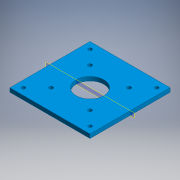
# Autodesk Inventor part: Part3
Saved by Autodesk Inventor 2016 (Build 200138000, 138)
## iProperties
Created: 2018-01-17
Part Number: Part3
Material: Generic
Document SubType Name: Modeling
Designer: student
Density: 1 g/cm^3
Appearance: Default
Author: student
Autodesk Inventor part; units mm, degrees
ref_plane "YZ Plane" through (0, 0, 0) normal (1, 0, 0) x (0, 1, 0)
ref_plane "XZ Plane" through (0, 0, 0) normal (0, 1, 0) x (-1, 0, 0)
ref_plane "XY Plane" through (0, 0, 0) normal (0, 0, 1) x (1, 0, 0)
sketch "Sketch1" plane through (0, 0, 0) normal (0, 1, 0) x (-1, 0, 0)
  circle A0 centre (86.3758, -99.5417) radius 1.5 projected
  circle A1 centre (117.3758, -99.5417) radius 1.5 projected
  circle A2 centre (117.3758, -130.5417) radius 1.5 projected
  circle A3 centre (86.3758, -130.5417) radius 1.5 projected
  circle A4 centre (101.8758, -115.0417) radius 11 projected
  line L0 (133.6258, -146.7917) -> (70.1258, -146.7917)
  line L1 (70.1258, -146.7917) -> (70.1258, -83.2917)
  line L2 (70.1258, -83.2917) -> (133.6258, -83.2917)
  line L3 (133.6258, -83.2917) -> (133.6258, -146.7917)
  line L4 (80.7258, -93.8917) -> (123.0258, -93.8917) construction
  line L5 (123.0258, -93.8917) -> (123.0258, -136.1917) construction
  line L6 (123.0258, -136.1917) -> (80.7258, -136.1917) construction
  line L7 (80.7258, -136.1917) -> (80.7258, -93.8917) construction
  line L8 (80.7258, -136.1917) -> (123.0258, -93.8917) construction
  line L9 (123.0258, -136.1917) -> (80.7258, -93.8917) construction
  circle A5 centre (75.4258, -88.5917) radius 1.4224
  circle A6 centre (75.4258, -141.4917) radius 1.4224
  circle A7 centre (128.3258, -141.4917) radius 1.4224
  circle A8 centre (128.3258, -88.5917) radius 1.4224
  point P0 (0, 0)
  dimension "d9" = 63.5
  dimension "d11" = 2.8448
  dimension "d12" = 2.8448
  dimension "d19" = 63.5
  dimension "d20" = 2.8448
  dimension "d21" = 2.8448
  constraints: 18 end point, 4 centre point, 3 perpendicular, 2 midpoint, 1 vertical
  measures "d9" distance of L0.end L1.end
  measures "d11" diameter of A5
  measures "d12" diameter of A6
  measures "d19" distance of L0.start L0.end
  measures "d20" diameter of A7
  measures "d21" diameter of A8
extrude "Extrusion1" add sketch "Sketch1" along normal blind 3.175
ref_plane "Work Plane1" through (-70.1258, 0, -115.0417) normal (0, 0, -1) x (-1, 0, 0)
body "Solid1"
